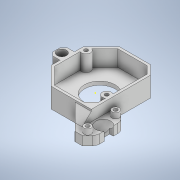
# Autodesk Inventor part: CameraMoldLogi
Saved by Autodesk Inventor 2020 (Build 240168000, 168)
## iProperties
Created: 2020-03-20
Part Number: CameraMoldLogi
Material: Generisch
Document SubType Name: Modeling
Designer: Fynn
Density: 1 g/cm^3
Appearance: Vorgabe
Author: Fynn
Autodesk Inventor part; units mm, degrees
ref_plane "YZ Plane" through (0, 0, 0) normal (1, 0, 0) x (0, 1, 0)
ref_plane "XZ Plane" through (0, 0, 0) normal (0, 1, 0) x (-1, 0, 0)
sketch "Skizze1" plane through (0, 0, 0) normal (0, 1, 0) x (-1, 0, 0)
  line L0 (-5.25, 27.5) -> (5.25, 27.5)
  line L1 (10.75, 22) -> (10.75, -22)
  line L2 (5.25, -27.5) -> (-5.25, -27.5)
  line L3 (-10.75, -22) -> (-10.75, 22)
  line L4 (-10.75, 27.5) -> (10.75, -27.5) construction
  line L5 (10.75, 27.5) -> (-10.75, -27.5) construction
  line L6 (10.75, 22) -> (5.25, 27.5)
  line L7 (10.75, -22) -> (5.25, -27.5)
  line L8 (-5.25, -27.5) -> (-10.75, -22)
  line L9 (-10.75, 22) -> (-5.25, 27.5)
  line L10 (7.25, 29.5) -> (-7.25, 29.5)
  line L11 (-12.75, 24) -> (-12.75, -24)
  line L12 (-7.25, -29.5) -> (7.25, -29.5)
  line L13 (12.75, -24) -> (12.75, 24)
  line L14 (12.75, 29.5) -> (-12.75, -29.5) construction
  line L15 (-12.75, 29.5) -> (12.75, -29.5) construction
  line L16 (12.75, 24) -> (7.25, 29.5)
  line L17 (12.75, -24) -> (7.25, -29.5)
  line L18 (-7.25, -29.5) -> (-12.75, -24)
  line L19 (-12.75, 24) -> (-7.25, 29.5)
  point P0 (0, 0)
  dimension "d0" = 21.5
  dimension "d1" = 55
  dimension "d2" = 5.5
  dimension "d3" = 5.5
  dimension "d4" = 5.5
  dimension "d5" = 5.5
  dimension "d6" = 5.5
  dimension "d7" = 5.5
  dimension "d8" = 5.5
  dimension "d9" = 5.5
  dimension "d10" = 2
  dimension "d11" = 2
  dimension "d12" = 5.5
  dimension "d13" = 5.5
  dimension "d14" = 5.5
  dimension "d15" = 5.5
  dimension "d16" = 5.5
  dimension "d17" = 5.5
  dimension "d18" = 5.5
  dimension "d19" = 5.5
  constraints: 40 end point, 16 point on line, 4 midpoint, 4 parallel, 2 horizontal, 2 perpendicular
  measures "d0" distance of L4.end L5.end
  measures "d1" distance of L5.start L4.end
  measures "d2" distance of L1.start L5.start
  measures "d3" distance of L0.end L5.start
  measures "d4" distance of L1.end L4.end
  measures "d5" distance of L2.start L4.end
  measures "d6" distance of L2.end L5.end
  measures "d7" distance of L3.start L5.end
  measures "d8" distance of L3.end L4.start
  measures "d9" distance of L0.start L4.start
  measures "d10" distance between parallel lines of L11 L3
  measures "d11" distance between parallel lines of L2 L12
  measures "d12" distance of L13.end L14.start
  measures "d13" distance of L10.start L14.start
  measures "d14" distance of L13.start L15.end
  measures "d15" distance of L12.end L15.end
  measures "d16" distance of L12.start L14.end
  measures "d17" distance of L11.end L14.end
  measures "d18" distance of L11.start L15.start
  measures "d19" distance of L10.end L15.start
extrude "Extrusion1" add sketch "Skizze1" along normal blind 10
sketch "Skizze3" plane through (0, 0, 0) normal (0, -1, 0) x (1, 0, 0)
  line L0 (7.25, -29.5) -> (-7.25, -29.5) projected
  line L1 (12.75, -24) -> (7.25, -29.5) projected
  line L2 (12.75, 24) -> (12.75, -24) projected
  line L3 (7.25, 29.5) -> (12.75, 24) projected
  line L4 (-7.25, 29.5) -> (7.25, 29.5) projected
  line L5 (-12.75, 24) -> (-7.25, 29.5) projected
  line L6 (-12.75, -24) -> (-12.75, 24) projected
  line L7 (-7.25, -29.5) -> (-12.75, -24) projected
  line L8 (-5.25, 27.5) -> (-10.75, 22) projected
  line L9 (5.25, 27.5) -> (-5.25, 27.5) projected
  line L10 (10.75, 22) -> (5.25, 27.5) projected
  line L11 (10.75, -22) -> (10.75, 22) projected
  line L12 (5.25, -27.5) -> (10.75, -22) projected
  line L13 (-5.25, -27.5) -> (5.25, -27.5) projected
  line L14 (-10.75, -22) -> (-5.25, -27.5) projected
  line L15 (-10.75, 22) -> (-10.75, -22) projected
  point P0 (0, 0)
extrude "Extrusion2" add sketch "Skizze3" along normal blind 2 contours L0 L7 L6 L5 L4 L3 L2 L1 | L9 L10 L11 L12 L13 L14 L15 L8
sketch "Skizze4" plane through (0, 0, 0) normal (0, 1, 0) x (1, 0, 0)
  line L0 (-10.75, -22) -> (-10.75, 22) projected
  line L1 (-10.75, -21) -> (-8.75, -21)
  line L2 (10.75, 22) -> (10.75, -22) projected
  line L3 (10.75, 18.3) -> (8.75, 18.3)
  circle A0 centre (-8.75, -21) radius 2
  circle A1 centre (8.75, 18.3) radius 2
  circle A2 centre (-8.75, -21) radius 0.55
  circle A3 centre (8.75, 18.3) radius 0.55
  point P0 (0, 0)
  dimension "d24" = 2
  dimension "d25" = 21
  dimension "d26" = 2
  dimension "d27" = 18.3
  dimension "d28" = 4
  dimension "d29" = 4
  dimension "d30" = 1.1
  dimension "d31" = 1.1
  constraints: 4 centre point, 4 coincident, 4 end point, 2 horizontal, 2 point on line
  measures "d24" distance of L1.start L1.end
  measures "d25" vertical distance of L1.start point (0, 0)
  measures "d26" distance of L3.start L3.end
  measures "d27" vertical distance of L3.start point (0, 0)
  measures "d28" diameter of A0
  measures "d29" diameter of A1
  measures "d30" diameter of A2
  measures "d31" diameter of A3
extrude "Extrusion3" add sketch "Skizze4" along normal blind 5
sketch "Skizze8" plane through (12.75, 10, 24) normal (1, 0, 0) x (0, 0, -1)
  line L0 (26.5, -23.1836) -> (21.5, -23.1836)
  line L1 (21.5, -23.1836) -> (21.5, 3.1836)
  line L2 (21.5, 3.1836) -> (26.5, 3.1836)
  line L3 (26.5, 3.1836) -> (26.5, -23.1836)
  line L4 (26.5, -23.1836) -> (21.5, 3.1836) construction
  line L5 (21.5, -23.1836) -> (26.5, 3.1836) construction
  point P0 (24, -10)
  dimension "d44" = 5
  constraints: 12 end point, 2 midpoint, 2 parallel, 1 horizontal, 1 perpendicular
  measures "d44" distance of L1.end L2.end
extrude "Extrusion7" cut sketch "Skizze8" against normal blind 8
sketch "Skizze9" plane through (0, -2, 0) normal (0, -1, 0) x (1, 0, 0)
  line L0 (4.75, -2.5) -> (4.75, 2.5) projected
  circle A0 centre (4.75, 0) radius 2.5
  point P0 (0, 0)
  point P1 (4.75, 2.5)
  constraints: 1 midpoint, 3 other
extrude "Extrusion8" cut sketch "Skizze9" against normal blind 12 contours A0 L0 picked at (4.3627, -0.7379)
sketch "Skizze17" plane through (0, 10, 0) normal (0, 1, 0) x (1, 0, 0)
  line L0 (6.25, -28) -> (-6.25, -28)
  line L1 (-11.25, -23) -> (-11.25, 23)
  line L2 (-6.25, 28) -> (6.25, 28)
  line L3 (11.25, 23) -> (11.25, -23)
  line L4 (11.25, -28) -> (-11.25, 28) construction
  line L5 (-11.25, -28) -> (11.25, 28) construction
  line L6 (-10.75, -22) -> (-10.75, 22) projected
  line L7 (5.25, -27.5) -> (-5.25, -27.5) projected
  line L8 (-11.25, -23) -> (-6.25, -28)
  line L9 (-11.25, 23) -> (-6.25, 28)
  line L10 (6.25, 28) -> (11.25, 23)
  line L11 (11.25, -23) -> (6.25, -28)
  line L12 (-5.25, -27.5) -> (-10.75, -22) projected
  line L13 (-10.75, 22) -> (-5.25, 27.5) projected
  line L14 (-5.25, 27.5) -> (5.25, 27.5) projected
  line L15 (5.25, 27.5) -> (10.75, 22) projected
  line L16 (10.75, 22) -> (10.75, 2.5) projected
  line L17 (10.75, -2.5) -> (10.75, -22) projected
  line L18 (10.75, -22) -> (5.25, -27.5) projected
  line L19 (12.75, -2.5) -> (10.75, -2.5) projected
  line L20 (10.75, -2.5) -> (10.75, 2.5)
  point P0 (0, 0)
  dimension "d74" = 0.5
  dimension "d75" = 0.5
  dimension "d80" = 5
  dimension "d81" = 5
  dimension "d82" = 5
  dimension "d83" = 5
  dimension "d84" = 5
  dimension "d85" = 5
  dimension "d86" = 5
  dimension "d87" = 5
  constraints: 22 end point, 12 point on line, 2 midpoint, 2 parallel, 2 perpendicular, 1 horizontal
  measures "d74" distance between parallel lines of L6 L1
  measures "d75" distance between parallel lines of L7 L0
  measures "d80" distance of L1.start point (-11.25, -28)
  measures "d81" distance of L0.end point (-11.25, -28)
  measures "d82" distance of L1.end L4.end
  measures "d83" distance of L2.start L4.end
  measures "d84" distance of L2.end L5.end
  measures "d85" distance of L3.start L5.end
  measures "d86" distance of L3.end L4.start
  measures "d87" distance of L0.start L4.start
extrude "Extrusion15" cut sketch "Skizze17" against normal up to surface (10 mm away)
sketch "Skizze18" plane through (12.75, -2, 24) normal (1, 0, 0) x (0, 0, -1)
  line L0 (21.5, 0) -> (21.5, 12) projected
  line L1 (0, 12) -> (21.5, 12) projected
  line L2 (0, 0) -> (0, 12) projected
  line L3 (21.5, 0) -> (0, 0) projected
  point P0 (24, 2)
extrude "Extrusion16" add sketch "Skizze18" along normal blind 10
ref_plane "Arbeitsebene1" through (0, 4, 0) normal (0, 1, 0) x (1, 0, 0)
sketch "Skizze19" plane through (0, 4, 0) normal (0, 1, 0) x (1, 0, 0)
  line L0 (12.75, -24) -> (7.25, -29.5) projected
  line L1 (4.75, -2.5) -> (22.75, -2.5) projected
  line L2 (12.75, -24) -> (22.75, -2.5)
  line L3 (22.75, -2.5) -> (22.75, -24) projected
  line L4 (22.75, -2.5) -> (22.75, -24)
  line L5 (22.75, -24) -> (12.75, -2.5)
  circle A0 centre (17.75, -13.25) radius 4.25
  line L6 (22, -13.25) -> (13.5, -13.25)
  point P0 (0, 0)
  dimension "d93" = 8.5
  constraints: 8 end point, 2 point on circle, 1 centre point, 1 collinear, 1 horizontal, 1 midpoint
  measures "d93" diameter of A0
revolve "Umdrehung1" cut sketch "Skizze19" angle 360 about axis through (22, 4, 13.25) along (-1, 0, 0) picked at (16.8466, -10.5822) picked at (14.953, -12.931) picked at (20.1235, -11.7363) contours A0 L2 L5 | L5 L6 A0 | A0 L6 L2
sketch "Skizze20" plane through (0, 10, 0) normal (0, 1, 0) x (1, 0, 0)
  line L0 (12.75, -24) -> (22.75, -24) projected
  line L1 (4.75, -2.5) -> (22.75, -2.5) projected
  line L2 (12.75, -24) -> (22.75, -2.5)
  line L3 (22.75, -2.5) -> (12.75, -2.5)
  line L4 (12.75, -24) -> (7.25, -29.5) projected
  line L5 (12.75, -24) -> (12.75, -2.5)
  line L6 (22.75, -2.5) -> (22.75, -24) projected
  point P0 (0, 0)
  constraints: 6 end point, 1 perpendicular, 1 point on line
extrude "Extrusion17" cut sketch "Skizze20" against normal blind 7
sketch "Skizze21" plane through (22.75, -2, 24) normal (1, 0, 0) x (0, 0, -1)
  line L0 (8.25, 12.4425) -> (13.25, 12.4425)
  line L1 (13.25, 12.4425) -> (13.25, -2.4425)
  line L2 (13.25, -2.4425) -> (8.25, -2.4425)
  line L3 (8.25, -2.4425) -> (8.25, 12.4425)
  line L4 (14.8807, 5) -> (6.6193, 5) projected
  line L5 (8.25, 12.4425) -> (13.25, -2.4425) construction
  line L6 (13.25, 12.4425) -> (8.25, -2.4425) construction
  point P0 (24, 2)
  point P1 (10.75, 5)
  point P2 (13.25, 5)
  point P3 (8.25, 5)
  dimension "d97" = 5
  constraints: 12 end point, 3 midpoint, 2 parallel, 1 horizontal, 1 perpendicular
  measures "d97" distance of L1.end L2.end
extrude "Extrusion18" cut sketch "Skizze21" against normal blind 4 contours L4 L1 L2 L3
sketch "Skizze22" plane through (22.75, -2, 24) normal (1, 0, 0) x (0, 0, -1)
  line L0 (-21.5, 10) -> (21.5, 10)
  line L1 (21.5, 10) -> (21.5, 0)
  line L2 (21.5, 0) -> (-21.5, 0)
  line L3 (-21.5, 0) -> (-21.5, 10)
  line L4 (-21.5, 10) -> (21.5, 0) construction
  line L5 (21.5, 10) -> (-21.5, 0) construction
  point P0 (24, 2)
  point P1 (0, 5)
  constraints: 12 end point, 2 midpoint, 2 parallel, 1 horizontal, 1 perpendicular
extrude "Extrusion19" cut sketch "Skizze22" against normal blind 2
sketch "Skizze23" plane through (0, 3, 0) normal (0, 1, 0) x (1, 0, 0)
  line L0 (20.75, -15.75) -> (20.75, -24) projected
  line L1 (12.75, -24) -> (12.75, -2.5) projected
  line L2 (20.75, -21) -> (16.75, -21)
  line L3 (16.75, -21) -> (16.75, -24)
  line L4 (12.75, -24) -> (20.75, -24) projected
  line L5 (20.75, -5.4005) -> (16.75, -5.4005)
  line L6 (16.75, -5.4005) -> (16.75, -2.4005)
  circle A0 centre (16.75, -21) radius 1.05
  circle A1 centre (16.75, -5.4005) radius 1.05
  point P0 (0, 0)
  dimension "d102" = 4
  dimension "d103" = 3
  dimension "d104" = 4
  dimension "d105" = 3
  dimension "d106" = 2.1
  dimension "d107" = 2.1
  constraints: 8 end point, 2 centre point, 2 coincident, 2 horizontal, 1 midpoint, 1 perpendicular, 1 point on line
  measures "d102" distance of L2.start L2.end
  measures "d103" distance of L2.end L3.end
  measures "d104" distance of L5.start L5.end
  measures "d105" distance of L5.end L6.end
  measures "d106" diameter of A0
  measures "d107" diameter of A1
extrude "Extrusion20" cut sketch "Skizze23" against normal through all contours A0 L3 L2 | L2 L3 A0 | A1 L6 L5 | L5 L6 A1
sketch "Skizze24" plane through (0, 3, 0) normal (0, 1, 0) x (1, 0, 0)
  point P0 (0, 0)
sketch "Skizze25" plane through (0, 3, 0) normal (0, 1, 0) x (1, 0, 0)
  circle A0 centre (16.75, -5.4005) radius 1.05 projected
  circle A1 centre (16.75, -5.4005) radius 2
  circle A2 centre (16.75, -21) radius 1.05 projected
  circle A3 centre (16.75, -21) radius 2
  point P0 (0, 0)
  dimension "d110" = 4
  dimension "d111" = 4
  constraints: 2 centre point, 2 coincident
  measures "d110" diameter of A1
  measures "d111" diameter of A3
extrude "Extrusion21" add sketch "Skizze25" along normal blind 3
sketch "Skizze26" plane through (0, 3, 0) normal (0, 1, 0) x (1, 0, 0)
  point P0 (0, 0)
chamfer "Fase2" distance 4 angle 45 2 edges at (20.75, 0.5, 2.5) (20.75, 0.5, 24)
fillet "Rundung2" radius 4 2 edges at (20.75, 0.5, 20) (20.75, 0.5, 6.5)
sketch "Skizze27" plane through (0, 10, 0) normal (0, 1, 0) x (1, 0, 0)
  line L0 (12.75, -24) -> (12.75, -2.5) projected
  line L1 (11.25, -2.5) -> (12.75, -2.5) projected
  line L2 (11.25, -2.5) -> (11.25, -23) projected
  line L3 (11.25, -23) -> (6.25, -28) projected
  line L4 (6.25, -28) -> (-6.25, -28) projected
  line L5 (-6.25, -28) -> (-11.25, -23) projected
  line L6 (-11.25, -23) -> (-11.25, 23) projected
  line L7 (-11.25, 23) -> (-6.25, 28) projected
  line L8 (-6.25, 28) -> (6.25, 28) projected
  line L9 (6.25, 28) -> (11.25, 23) projected
  line L10 (11.25, 23) -> (11.25, 2.5) projected
  line L11 (11.25, 2.5) -> (12.75, 2.5) projected
  line L12 (12.75, 2.5) -> (12.75, 24) projected
  line L13 (12.75, 24) -> (7.25, 29.5) projected
  line L14 (7.25, 29.5) -> (-7.25, 29.5) projected
  line L15 (-7.25, 29.5) -> (-12.75, 24) projected
  line L16 (-12.75, 24) -> (-12.75, -24) projected
  line L17 (-12.75, -24) -> (-7.25, -29.5) projected
  line L18 (-7.25, -29.5) -> (7.25, -29.5) projected
  line L19 (7.25, -29.5) -> (12.75, -24) projected
  circle A0 centre (-8.75, -21) radius 2 projected
  circle A1 centre (8.75, 18.3) radius 2 projected
  circle A2 centre (8.75, 18.3) radius 0.55 projected
  point P0 (0, 0)
extrude "Extrusion22" cut sketch "Skizze27" against normal up to surface (10 mm away) contours L19 L18 L17 L16 L15 L14 L13 L12 L11 L10 L9 L8 L7 L6 L5 L4 L3 L2 L1 L0 | A0 | A1 | A2
sketch "Skizze28" plane through (0, 0, 0) normal (0, 1, 0) x (1, 0, 0)
  circle A0 centre (10, -3.6) radius 2.5
  circle A1 centre (10, -3.6) radius 1.05
  circle A2 centre (-13, 11.7) radius 2.5
  circle A3 centre (-13, 11.7) radius 1.05
  point P0 (0, 0)
  dimension "d120" = 3.6
  dimension "d121" = 10
  dimension "d122" = 5
  dimension "d123" = 2.1
  dimension "d124" = 13
  dimension "d125" = 11.7
  dimension "d126" = 2.1
  dimension "d127" = 5
  constraints: 5 coincident, 4 centre point
  measures "d120" vertical distance of point (10, -3.6) point (0, 0)
  measures "d121" horizontal distance of point (10, -3.6) point (0, 0)
  measures "d122" diameter of A0
  measures "d123" diameter of A1
  measures "d124" horizontal distance of point (-13, 11.7) point (0, 0)
  measures "d125" vertical distance of point (-13, 11.7) point (0, 0)
  measures "d126" diameter of A3
  measures "d127" diameter of A2
extrude "Extrusion23" add sketch "Skizze28" along normal blind 9
sketch "Skizze29" plane through (0, 0, 0) normal (0, 1, 0) x (1, 0, 0)
  line L0 (12.75, 2.5) -> (4.75, 2.5) projected
  line L1 (4.75, -2.5) -> (7.755, -2.5) projected
  line L2 (12.75, -2.5) -> (16.75, -2.5) projected
  line L3 (4.75, -2.5) -> (16.75, -2.5) projected
  line L4 (4.75, -2.5) -> (7.755, -2.5) projected
  line L5 (7.755, -2.5) -> (12.245, -2.5) projected
  line L6 (12.245, -2.5) -> (12.75, -2.5) projected
  arc A0 (4.75, 2.5) -> (4.75, -2.5) centre (4.75, 0) ccw projected
  line L7 (12.75, 2.5) -> (12.75, -2.5)
  point P0 (0, 0)
  constraints: 2 end point, 1 vertical
extrude "Extrusion24" add sketch "Skizze29" against normal up to surface (2 mm away)
sketch "Skizze30" plane through (0, 0, 0) normal (0, 1, 0) x (1, 0, 0)
  arc A0 (-12.75, 12.7198) -> (-12.75, 10.6802) centre (-13, 11.7) ccw projected
  circle A1 centre (10, -3.6) radius 1.05 projected
  line L0 (-13, 11.7) -> (10, -3.6)
  line L1 (-13, 11.7) -> (6.15, 11.7)
  line L2 (10, -3.6) -> (-13, -3.6)
  line L3 (-12.75, -24) -> (-12.75, 24) projected
  line L4 (-13, 11.7) -> (-13, -3.6)
  line L5 (6.15, 11.7) -> (-13, -3.6)
  line L6 (12.75, -14.95) -> (-9.6, -14.95)
  line L7 (-19.6, -4.95) -> (-19.6, 13.05)
  line L8 (-9.6, 23.05) -> (7.75, 23.05)
  line L9 (12.75, 18.05) -> (12.75, -14.95)
  line L10 (12.75, -14.95) -> (-19.6, 23.05) construction
  line L11 (-19.6, -14.95) -> (12.75, 23.05) construction
  line L12 (12.75, -2.5) -> (12.75, 24) projected
  line L13 (-19.6, 13.05) -> (-9.6, 23.05)
  line L14 (-19.6, -4.95) -> (-9.6, -14.95)
  line L15 (12.75, 18.05) -> (7.75, 23.05)
  point P0 (0, 0)
  point P1 (-3.425, 4.05)
  dimension "d132" = 38
  dimension "d133" = 29.6
  dimension "d134" = 10
  dimension "d135" = 10
  dimension "d136" = 10
  dimension "d137" = 10
  dimension "d138" = 5
  dimension "d139" = 5
  constraints: 28 end point, 6 point on line, 3 midpoint, 2 horizontal, 2 parallel, 2 perpendicular, 1 collinear, 1 vertical
  measures "d132" distance between parallel lines of L6 L8
  measures "d133" distance from line of L0.end L7
  measures "d134" distance of L7.end L10.end
  measures "d135" distance of L8.start L10.end
  measures "d136" distance of L7.start L11.start
  measures "d137" distance of L6.end L11.start
  measures "d138" distance of L9.start L11.end
  measures "d139" distance of L8.end L11.end
extrude "Extrusion25" add sketch "Skizze30" against normal blind 5 contours L3 L13 L8 L15 L9 L6 L14 L2 A1 L0 L5 L1 | A0 L4 L2 L3 L14 L7 L13 | A0 L3 L5 L4 | L1 L5 L0 L3 | L3 L0 L5 | L5 L3 L2 | L5 L0 A1 L2 L3
sketch "Skizze31" plane through (0, -2, 0) normal (0, -1, 0) x (1, 0, 0)
  line L0 (12.75, -18.05) -> (7.75, -23.05) projected
  line L1 (7.75, -23.05) -> (-9.6, -23.05) projected
  line L2 (-9.6, -23.05) -> (-12.75, -19.9) projected
  line L3 (-12.75, -19.9) -> (-12.75, -24) projected
  line L4 (-12.75, -24) -> (-7.25, -29.5) projected
  line L5 (-7.25, -29.5) -> (7.25, -29.5) projected
  line L6 (7.25, -29.5) -> (12.75, -24) projected
  line L7 (12.75, -18.05) -> (12.75, -24) projected
  line L8 (12.75, 24) -> (12.75, 2.5) projected
  line L9 (12.75, 14.95) -> (12.75, 2.5) projected
  line L10 (12.75, 2.5) -> (16.75, 2.5) projected
  line L11 (19.5784, 5.3284) -> (16.75, 2.5) projected
  arc A0 (19.5784, 5.3284) -> (20.75, 8.1569) centre (16.75, 8.1569) ccw projected
  line L12 (20.75, 8.1569) -> (20.75, 10.75) projected
  line L13 (20.75, 10.75) -> (18.75, 10.75) projected
  line L14 (18.75, 10.75) -> (18.75, 15.75) projected
  line L15 (18.75, 15.75) -> (20.75, 15.75) projected
  line L16 (20.75, 15.75) -> (20.75, 18.3431) projected
  arc A1 (20.75, 18.3431) -> (19.5784, 21.1716) centre (16.75, 18.3431) ccw projected
  line L17 (16.75, 24) -> (19.5784, 21.1716) projected
  line L18 (12.75, 24) -> (16.75, 24) projected
  line L19 (12.75, 24) -> (7.25, 29.5) projected
  line L20 (7.25, 29.5) -> (-7.25, 29.5) projected
  line L21 (-7.25, 29.5) -> (-12.75, 24) projected
  line L22 (-12.75, 24) -> (-12.75, 11.8) projected
  line L23 (-12.75, 11.8) -> (-9.6, 14.95) projected
  line L24 (-9.6, 14.95) -> (12.75, 14.95) projected
  circle A2 centre (16.75, 21) radius 1.05 projected
  circle A3 centre (16.75, 5.4005) radius 1.05 projected
  point P0 (0, 0)
extrude "Extrusion26" cut sketch "Skizze31" against normal through all contours L7 L6 L5 L4 L3 L2 L1 L0 | L8 L24 L23 L22 L21 L20 L19
sketch "Skizze32" plane through (-13, 9, -11.7) normal (0, 1, 0) x (1, 0, 0)
  circle A0 centre (0, 0) radius 1.05 projected
  circle A1 centre (23, -15.3) radius 1.05 projected
  point P0 (13, -11.7)
extrude "Extrusion27" cut sketch "Skizze32" against normal through all
sketch "Skizze33" plane through (0, 0, 0) normal (0, 1, 0) x (1, 0, 0)
  circle A0 centre (-13, 11.7) radius 1.05 projected
  circle A1 centre (10, -3.6) radius 1.05 projected
  line L0 (-13, 11.7) -> (10, -3.6)
  line L1 (-13, 11.7) -> (-13, -3.6)
  line L2 (-13, -3.6) -> (10, 11.7)
  circle A2 centre (-1.5, 4.05) radius 8.5
  point P0 (0, 0)
  dimension "d146" = 17
  constraints: 6 end point, 1 centre point, 1 midpoint, 1 vertical
  measures "d146" diameter of A2
extrude "Extrusion28" cut sketch "Skizze33" against normal through all contours A2 L2 L0 | L0 L2 A2 | L2 L0 A2 | L2 A2 L0
sketch "Skizze34" plane through (0, 0, 0) normal (0, 1, 0) x (1, 0, 0)
  circle A0 centre (-1.5, 4.05) radius 8.5 projected
  line L0 (-19.6, -4.95) -> (-9.6, -14.95) projected
  line L1 (-9.6, -14.95) -> (12.75, -14.95) projected
  line L2 (12.75, -14.95) -> (12.75, -2.5) projected
  line L3 (12.75, -2.5) -> (12.75, 18.05) projected
  line L4 (12.75, 18.05) -> (7.75, 23.05) projected
  line L5 (7.75, 23.05) -> (-9.6, 23.05) projected
  line L6 (-9.6, 23.05) -> (-19.6, 13.05) projected
  line L7 (-19.6, 13.05) -> (-19.6, -4.95) projected
  circle A1 centre (10, -3.6) radius 2.5 projected
  circle A2 centre (-13, 11.7) radius 2.5 projected
  line L8 (12.75, -14.95) -> (12.75, -2.5) projected
  line L9 (7.925, -13.55) -> (-9.0201, -13.55)
  line L10 (-9.0201, -13.55) -> (-18.2, -4.3701)
  line L11 (-18.2, -4.3701) -> (-18.2, 12.4701)
  line L12 (-19.6, -4.95) -> (-19.6, 13.05) projected
  line L13 (-18.2, 12.4701) -> (-9.3936, 21.2765)
  line L14 (7.1701, 21.65) -> (11.35, 17.4701)
  line L15 (11.35, 17.4701) -> (11.35, -10.125)
  line L16 (-9.0201, 21.65) -> (7.1701, 21.65)
  line L17 (-9.3936, 21.2765) -> (-9.0201, 21.65)
  line L18 (7.1701, -13.55) -> (11.35, -9.3701)
  point P0 (0, 0)
  point P1 (11.35, -1.4958)
  point P2 (11.35, -5.7042)
  dimension "d149" = 1.4
  dimension "d150" = 1.4
  dimension "d151" = 1.4
  dimension "d152" = 1.4
  dimension "d153" = 1.4
  dimension "d154" = 1.4
  dimension "d155" = 1.4
  constraints: 18 end point, 4 parallel, 2 point on line, 1 horizontal, 1 perpendicular
  measures "d149" distance between parallel lines of L11 L7
  measures "d150" distance between parallel lines of L6 L13
  measures "d151" distance between parallel lines of L5 L16
  measures "d152" distance between parallel lines of L4 L14
  measures "d153" distance between parallel lines of L3 L15
  measures "d154" distance between parallel lines of L1 L9
  measures "d155" distance between parallel lines of L0 L10
extrude "Extrusion29" add sketch "Skizze34" along normal blind 9 contours L7 L6 L5 L4 L3 L2 L1 L0
sketch "Skizze35" plane through (0, -2, 0) normal (0, -1, 0) x (1, 0, 0)
  circle A0 centre (-1.5, -4.05) radius 8.5 projected
  circle A1 centre (-13, -11.7) radius 1.05 projected
  line L0 (-9.6, -23.05) -> (7.75, -23.05) projected
  line L1 (7.75, -23.05) -> (12.75, -18.05) projected
  line L2 (12.75, -18.05) -> (12.75, 14.95) projected
  line L3 (12.75, 14.95) -> (-9.6, 14.95) projected
  line L4 (-9.6, 14.95) -> (-19.6, 4.95) projected
  line L5 (-19.6, 4.95) -> (-19.6, -13.05) projected
  line L6 (-19.6, -13.05) -> (-9.6, -23.05) projected
  circle A2 centre (10, 3.6) radius 1.05 projected
  point P0 (0, 0)
extrude "Extrusion30" cut sketch "Skizze35" along normal blind 9
sketch "Skizze36" plane through (-13, 9, -11.7) normal (0, 1, 0) x (1, 0, 0)
  circle A0 centre (0, 0) radius 2.5 projected
  circle A1 centre (0, 0) radius 1.05 projected
  point P0 (13, -11.7)
extrude "Extrusion31" cut sketch "Skizze36" against normal up to surface (9 mm away)
sketch "Skizze37" plane through (0, 0, 0) normal (0, 1, 0) x (1, 0, 0)
  circle A0 centre (-13, 11.7) radius 1.05 projected
  point P0 (0, 0)
extrude "Extrusion32" add sketch "Skizze37" against normal up to surface (2 mm away)
sketch "Skizze38" plane through (0, 0, 0) normal (0, 1, 0) x (1, 0, 0)
  circle A0 centre (-17.15, 12.0352) radius 1.05
  line L0 (-18.2, 12.4701) -> (-9.0201, 21.65) projected
  line L1 (-18.2, -4.3701) -> (-18.2, 12.4701) projected
  point P0 (0, 0)
  dimension "d164" = 2.1
  dimension "d165" = 1.05
  dimension "d166" = 1.05
  constraints: 1 centre point, 1 coincident
  measures "d164" diameter of A0
  measures "d165" distance from line of L0 A0.centre
  measures "d166" distance from line of L1 A0.centre
extrude "Extrusion33" cut sketch "Skizze38" against normal through all contours A0
sketch "Skizze39" plane through (0, 0, 0) normal (0, 1, 0) x (1, 0, 0)
  arc A0 (-18.2, 12.0352) -> (-17.8925, 12.7776) centre (-17.15, 12.0352) ccw projected
  line L0 (-19.6, -4.95) -> (-9.6, -14.95) projected
  line L1 (-9.6, -14.95) -> (12.75, -14.95) projected
  line L2 (12.75, -14.95) -> (12.75, 18.05) projected
  line L3 (12.75, 18.05) -> (7.75, 23.05) projected
  line L4 (7.75, 23.05) -> (-9.6, 23.05) projected
  line L5 (-9.6, 23.05) -> (-19.6, 13.05) projected
  line L6 (-19.6, 13.05) -> (-19.6, -4.95) projected
  arc A1 (11.35, -1.4958) -> (11.35, -5.7042) centre (10, -3.6) ccw projected
  line L7 (11.35, -5.7042) -> (11.35, -9.3701) projected
  line L8 (11.35, -9.3701) -> (7.1701, -13.55) projected
  line L9 (7.1701, -13.55) -> (-9.0201, -13.55) projected
  line L10 (-9.0201, -13.55) -> (-18.2, -4.3701) projected
  line L11 (-18.2, -4.3701) -> (-18.2, 12.4701) projected
  line L12 (-18.2, 12.4701) -> (-9.0201, 21.65) projected
  line L13 (-9.0201, 21.65) -> (7.1701, 21.65) projected
  line L14 (7.1701, 21.65) -> (11.35, 17.4701) projected
  line L15 (11.35, 17.4701) -> (11.35, -1.4958) projected
  circle A2 centre (10, -3.6) radius 1.05 projected
  arc A3 (-18.2, 9.7664) -> (-16.2882, 14.3819) centre (-17.15, 12.0352) ccw
  arc A4 (-19.2342, 13.4158) -> (-19.6, 12.5327) centre (-17.15, 12.0352) ccw
  point P0 (0, 0)
  constraints: 4 point on circle, 4 point on line, 2 centre point, 1 coincident
extrude "Extrusion34" add sketch "Skizze39" along normal up to surface (9 mm away) contours L11 L12 A0 | A0 L12 A3 L11
sketch "Skizze40" plane through (-17.15, 0, -12.0352) normal (0, -1, 0) x (1, 0, 0)
  circle A0 centre (0, 0) radius 1.05 projected
  point P0 (17.15, 12.0352)
extrude "Extrusion35" cut sketch "Skizze40" against normal through all
sketch "Skizze41" plane through (0, -2, 0) normal (0, -1, 0) x (1, 0, 0)
  circle A0 centre (-22.6, -4.05) radius 2.5
  line L0 (-19.6, -13.05) -> (-19.6, 4.95) projected
  line L1 (-19.6, -8.05) -> (-25.6, -8.05)
  line L2 (-25.6, -8.05) -> (-25.6, -0.05)
  line L3 (-25.6, -0.05) -> (-19.6, -0.05)
  line L4 (-19.6, -0.05) -> (-19.6, -8.05)
  point P0 (0, 0)
  dimension "d174" = 5
  dimension "d175" = 3
  dimension "d177" = 4
  dimension "d178" = 4
  dimension "d179" = 3
  constraints: 8 end point, 2 parallel, 1 centre point, 1 horizontal, 1 perpendicular, 1 point on line
  measures "d174" diameter of A0
  measures "d175" distance from line of L0 A0.centre
  measures "d177" distance from line of L1 A0.centre
  measures "d178" distance from line of A0.centre L3
  measures "d179" distance from line of A0.centre L2
extrude "Extrusion36" add sketch "Skizze41" against normal blind 5
chamfer "Fase3" distance 2 angle 45 2 edges at (-25.6, 0.5, -8.05) (-25.6, 0.5, -0.05)
chamfer "Fase4" distance 9 angle 45 1 edges at (12.75, 0.5, 14.95)
chamfer "Fase5" distance 5 angle 45 1 edges at (8.25, 3, 14.95)
sketch "Skizze42" plane through (0, 3, 0) normal (0, 1, 0) x (1, 0, 0)
  line L0 (-23.6, 0.05) -> (-25.6, 2.05) projected
  line L1 (-23.6, 0.05) -> (-19.6, 0.05) projected
  line L2 (-19.6, 8.05) -> (-19.6, 0.05) projected
  line L3 (-19.6, 8.05) -> (-23.6, 8.05) projected
  line L4 (-25.6, 6.05) -> (-23.6, 8.05) projected
  line L5 (-25.6, 6.05) -> (-25.6, 2.05) projected
  circle A0 centre (-22.6, 4.05) radius 2.5 projected
  point P0 (0, 0)
extrude "Extrusion37" add sketch "Skizze42" along normal up to surface (6 mm away)
sketch "Skizze43" plane through (0, -2, 0) normal (0, -1, 0) x (1, 0, 0)
  circle A0 centre (-22.6, -4.05) radius 2.5 projected
  circle A1 centre (-17.15, -12.0352) radius 1.05 projected
  circle A2 centre (10, 3.6) radius 1.05 projected
  circle A3 centre (-1.5, -4.05) radius 8.5 projected
  line L0 (-25.6, -2.05) -> (-23.6, -0.05) projected
  line L1 (-25.6, -2.05) -> (-25.6, -6.05) projected
  line L2 (-23.6, -8.05) -> (-25.6, -6.05) projected
  line L3 (-23.6, -8.05) -> (-19.6, -8.05) projected
  line L4 (-19.6, -13.05) -> (-19.6, -8.05) projected
  line L5 (-9.6, -23.05) -> (-19.6, -13.05) projected
  line L6 (7.75, -23.05) -> (-9.6, -23.05) projected
  line L7 (12.75, -18.05) -> (7.75, -23.05) projected
  line L8 (12.75, 2.5) -> (12.75, -18.05) projected
  line L9 (12.75, 2.5) -> (16.75, 2.5) projected
  line L10 (19.5784, 5.3284) -> (16.75, 2.5) projected
  arc A4 (19.5784, 5.3284) -> (20.75, 8.1569) centre (16.75, 8.1569) ccw projected
  line L11 (20.75, 8.1569) -> (20.75, 10.75) projected
  line L12 (20.75, 10.75) -> (18.75, 10.75) projected
  line L13 (18.75, 10.75) -> (18.75, 15.75) projected
  line L14 (18.75, 15.75) -> (20.75, 15.75) projected
  line L15 (20.75, 15.75) -> (20.75, 18.3431) projected
  arc A5 (20.75, 18.3431) -> (19.5784, 21.1716) centre (16.75, 18.3431) ccw projected
  line L16 (16.75, 24) -> (19.5784, 21.1716) projected
  line L17 (12.75, 24) -> (16.75, 24) projected
  line L18 (12.75, 24) -> (12.75, 23.95) projected
  line L19 (3.75, 14.95) -> (12.75, 23.95) projected
  line L20 (-9.6, 14.95) -> (3.75, 14.95) projected
  line L21 (-19.6, 4.95) -> (-9.6, 14.95) projected
  line L22 (-19.6, -0.05) -> (-19.6, 4.95) projected
  line L23 (-19.6, -0.05) -> (-23.6, -0.05) projected
  circle A6 centre (16.75, 21) radius 1.05 projected
  circle A7 centre (16.75, 5.4005) radius 1.05 projected
  line L24 (-19.6, -13.05) -> (-19.6, -8.05) projected
  line L25 (-19.6, -0.05) -> (-19.6, 4.95) projected
  line L26 (-19.6, -8.05) -> (-19.6, -0.05)
  point P0 (0, 0)
  constraints: 2 end point, 1 collinear
extrude "Extrusion38" cut sketch "Skizze43" against normal blind 6 contours L0 L23 L26 L3 L2 L1
sketch "Skizze44" plane through (0, 9, 0) normal (0, 1, 0) x (1, 0, 0)
  circle A0 centre (-22.6, 4.05) radius 2.5 projected
  point P0 (0, 0)
  constraints: 1 coincident
hole "Bohrung1" at (-22.6, 9, -4.05) direction (0, -1, 0) diameter 5.2 end through all
equation "\"d3\" = d2"
equation "\"d5\" = d4"
equation "\"d6\" = d4"
equation "\"d7\" = d6"
equation "\"d8\" = d4"
equation "\"d9\" = d8"
equation "\"d13\" = d12"
equation "\"d14\" = d12"
equation "\"d15\" = d14"
equation "\"d16\" = d12"
equation "\"d17\" = d16"
equation "\"d18\" = d12"
equation "\"d19\" = d18"
equation "\"d81\" = d80"
equation "\"d83\" = d82"
equation "\"d84\" = d82"
equation "\"d85\" = d84"
equation "\"d86\" = d82"
equation "\"d87\" = d86"
equation "\"d135\" = d134"
equation "\"d136\" = d134"
equation "\"d137\" = d136"
equation "\"d139\" = d138"
